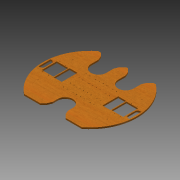
# Autodesk Inventor part: ChassisRound
Saved by Autodesk Inventor 2014 SP1 (Build 180222100, 222)
## iProperties
Created: 2015-03-16
Part Number: ChassisRound
Material: Wood (Oak)
Document SubType Name: Modeling
Designer: david
Density: 0.76 g/cm^3
Appearance: Yellow Pine - Solid Stained Light Low Gloss
Mass: 358.304 g
Surface Area: 1717.54 cm^2
Volume: 471.453 cm^3
Chassis_Body_Length: 300,000 mm
Chassis_Body_Diameter: 380,000 mm
Chassis_Body_Thickness: 6,000 mm
Author: david
Autodesk Inventor part; units mm, degrees
ref_plane "YZ Plane" through (0, 0, 0) normal (1, 0, 0) x (0, 1, 0)
ref_plane "XZ Plane" through (0, 0, 0) normal (0, 1, 0) x (-1, 0, 0)
ref_plane "XY Plane" through (0, 0, 0) normal (0, 0, 1) x (1, 0, 0)
sketch "BodySketch" plane through (0, 0, 0) normal (0, 1, 0) x (-1, 0, 0)
  line L0 (0, 150) -> (116.619, 150)
  line L1 (116.619, -150) -> (0, -150)
  line L2 (0, 0) -> (0, 145.614) construction
  line L3 (0, 150) -> (-116.619, 150)
  line L4 (-116.619, -150) -> (0, -150)
  line L5 (0, 0) -> (316.974, 0) construction
  arc A0 (116.619, -150) -> (116.619, 150) centre (0, 0) ccw
  arc A1 (-116.619, 150) -> (-116.619, -150) centre (0, 0) ccw
  dimension "Chassis_Body_Length" = 300
  dimension "d76" = 190
  constraints: 12 end point, 4 point on circle, 3 parallel, 2 centre point, 2 point on line, 2 symmetric about line, 1 coincident, 1 horizontal, 1 perpendicular, 1 other
  measures "Chassis_Body_Length" distance between parallel lines of L1 L0
  measures "d76" radius of A0
extrude "Body" add sketch "BodySketch" along normal blind 6
sketch "EncoderWheelHoleSketch" plane through (0, 6, 0) normal (0, 1, 0) x (1, 0, 0)
  line L0 (-168.5, 18) -> (-168.5, -18)
  line L1 (-184, -24.5) -> (-184, 24.5)
  line L2 (-116.619, -150) -> (116.619, -150) projected
  arc A0 (-116.619, 150) -> (-116.619, -150) centre (0, 0) ccw projected
  line L3 (-184, 24.5) -> (-177, 24.5)
  line L4 (-177, 24.5) -> (-168.5, 18)
  line L5 (-168.5, -18) -> (-177, -24.5)
  line L6 (-177, -24.5) -> (-184, -24.5)
  line L7 (0, 0) -> (-101.7765, 0) construction
  line L8 (0, 0) -> (0, 68.8757) construction
  line L9 (168.5, 18) -> (168.5, -18)
  line L10 (184, -24.5) -> (184, 24.5)
  line L11 (184, 24.5) -> (177, 24.5)
  line L12 (177, 24.5) -> (168.5, 18)
  line L13 (168.5, -18) -> (177, -24.5)
  line L14 (177, -24.5) -> (184, -24.5)
  point P0 (-190, 0)
  dimension "d80" = 7
  dimension "d81" = 15.5
  dimension "d82" = 49
  dimension "d83" = 36
  dimension "d84" = 6
  constraints: 28 end point, 7 symmetric about line, 5 parallel, 1 perpendicular, 1 point on circle, 1 point on line, 1 other
  measures "d80" distance of L1.end L3.end
  measures "d81" distance between parallel lines of L0 L1
  measures "d82" distance between parallel lines of L6 L3
  measures "d83" distance of L0.start L0.end
  measures "d84" distance from line of point (-190, 0) L1
extrude "EncoderWheelHole" cut sketch "EncoderWheelHoleSketch" against normal up to next
sketch "EncoderBodyHoleSketch" plane through (0, 6, 0) normal (0, 1, 0) x (1, 0, 0)
  line L0 (0, 0) -> (0, 145.3586) construction
  line L1 (-164.5, 30.25) -> (-117.5, 30.25)
  line L2 (-117.5, 30.25) -> (-117.5, -30.25)
  line L3 (-117.5, -30.25) -> (-164.5, -30.25)
  line L4 (-164.5, -30.25) -> (-164.5, 30.25)
  line L5 (0, 0) -> (187.4589, 0) construction
  line L6 (164.5, 30.25) -> (117.5, 30.25)
  line L7 (117.5, 30.25) -> (117.5, -30.25)
  line L8 (117.5, -30.25) -> (164.5, -30.25)
  line L9 (164.5, -30.25) -> (164.5, 30.25)
  line L10 (-141, -22.1441) -> (-141, 50.5352) construction
  line L11 (-168.5, 18) -> (-168.5, -18) projected
  line L12 (-184, -24.5) -> (-184, 24.5) projected
  dimension "d9" = 47
  dimension "d10" = 60.5
  dimension "d85" = 43
  constraints: 22 end point, 4 symmetric about line, 3 parallel, 2 perpendicular, 1 horizontal, 2 other
  measures "d9" distance between parallel lines of L2 L4
  measures "d10" distance between parallel lines of L3 L1
  measures "d85" distance between parallel lines of L12 L10
extrude "EncoderBodyHole" cut sketch "EncoderBodyHoleSketch" against normal up to next
sketch "EncoderSupportFasteningSketch" plane through (0, 6, 0) normal (0, 1, 0) x (1, 0, 0)
  line L0 (-128.5, 39.75) -> (-161.5, 39.75) construction
  line L1 (-161.5, 39.75) -> (-161.5, -39.75) construction
  line L2 (-128.5, -39.75) -> (-128.5, 39.75) construction
  circle A0 centre (-156.5, 34.75) radius 1.5
  line L3 (-145, 46.4919) -> (-145, -51.9033) construction
  circle A1 centre (-133.5, 34.75) radius 1.5
  line L4 (0, 0) -> (78.2402, 0) construction
  circle A2 centre (-156.5, -34.75) radius 1.5
  circle A3 centre (-133.5, -34.75) radius 1.5
  line L5 (-161.5, -39.75) -> (-128.5, -39.75) construction
  line L6 (0, 0) -> (0, 64.4845) construction
  circle A4 centre (156.5, 34.75) radius 1.5
  circle A5 centre (133.5, 34.75) radius 1.5
  circle A6 centre (156.5, -34.75) radius 1.5
  circle A7 centre (133.5, -34.75) radius 1.5
  line L7 (-184, -24.5) -> (-184, 24.5) projected
  dimension "d17" = 33
  dimension "d19" = 3
  dimension "d20" = 5
  dimension "d21" = 5
  dimension "d22" = 16.5
  dimension "d69" = 79.5
  dimension "d86" = 22.5
  constraints: 14 end point, 8 centre point, 7 symmetric about line, 2 parallel, 2 perpendicular, 1 horizontal, 8 other
  measures "d17" distance between parallel lines of L1 L2
  measures "d19" diameter of A0
  measures "d20" distance from line of L0 A0.centre
  measures "d21" distance from line of L1 A0.centre
  measures "d22" distance between parallel lines of L1 L3
  measures "d69" distance between parallel lines of L5 L0
  measures "d86" distance between parallel lines of L7 L1
extrude "EncoderSupportFastening" cut sketch "EncoderSupportFasteningSketch" against normal up to next
sketch "MotorBlockFasteningSketch" plane through (0, 6, 0) normal (0, 1, 0) x (1, 0, 0)
  line L0 (10.676, -18) -> (24.3135, -18) construction
  circle A0 centre (7.5, -18) radius 1.5
  circle A1 centre (22.5, -18) radius 1.5
  line L1 (0, 0) -> (0, -28.6489) construction
  circle A2 centre (46.5, -18) radius 1.5
  circle A3 centre (61.5, -18) radius 1.5
  circle A4 centre (7.5, -46) radius 1.5
  circle A5 centre (22.5, -46) radius 1.5
  circle A6 centre (46.5, -46) radius 1.5
  circle A7 centre (61.5, -46) radius 1.5
  circle A8 centre (-7.5, -18) radius 1.5
  circle A9 centre (-22.5, -18) radius 1.5
  circle A10 centre (-46.5, -18) radius 1.5
  circle A11 centre (-61.5, -18) radius 1.5
  circle A12 centre (-7.5, -46) radius 1.5
  circle A13 centre (-22.5, -46) radius 1.5
  circle A14 centre (-46.5, -46) radius 1.5
  circle A15 centre (-61.5, -46) radius 1.5
  line L2 (0, 0) -> (72.0385, 0) construction
  circle A16 centre (7.5, 18) radius 1.5
  circle A17 centre (22.5, 18) radius 1.5
  line L3 (0, 0) -> (0, 28.6489) construction
  circle A18 centre (46.5, 18) radius 1.5
  circle A19 centre (61.5, 18) radius 1.5
  circle A20 centre (7.5, 46) radius 1.5
  circle A21 centre (22.5, 46) radius 1.5
  circle A22 centre (46.5, 46) radius 1.5
  circle A23 centre (61.5, 46) radius 1.5
  circle A24 centre (-7.5, 18) radius 1.5
  circle A25 centre (-22.5, 18) radius 1.5
  circle A26 centre (-46.5, 18) radius 1.5
  circle A27 centre (-46.5, 46) radius 1.5
  circle A28 centre (-61.5, 18) radius 1.5
  circle A29 centre (-61.5, 46) radius 1.5
  circle A30 centre (-7.5, 46) radius 1.5
  circle A31 centre (-22.5, 46) radius 1.5
  dimension "d25" = 3
  dimension "d28" = 15
  dimension "d35" = 39
  dimension "d38" = 28
  dimension "d41" = 15
  dimension "d46" = 18
  constraints: 32 centre point, 25 symmetric about line, 8 end point, 3 horizontal, 1 perpendicular, 1 point on line, 1 vertical, 38 other
  measures "d25" diameter of A0
  measures "d28" distance of A0.centre A1.centre
  measures "d35" distance of A0.centre A2.centre
  measures "d38" distance of A0.centre A4.centre
  measures "d41" distance of A0.centre A8.centre
  measures "d46" distance between parallel lines of L2 L0
extrude "MotorBlockFastening" cut sketch "MotorBlockFasteningSketch" against normal up to next
sketch "MotorWheelHoleSketch" plane through (0, 6, 0) normal (0, 1, 0) x (1, 0, 0)
  line L0 (-114.5, 32) -> (-82.5, 32)
  line L1 (-82.5, 32) -> (-82.5, -32)
  line L2 (-82.5, -32) -> (-114.5, -32)
  line L3 (-114.5, -32) -> (-114.5, 32)
  line L4 (0, 0) -> (64.8732, 0) construction
  line L5 (0, 0) -> (0, 63.2492) construction
  line L6 (-117.5, 30.25) -> (-117.5, -30.25) construction
  line L7 (114.5, 32) -> (82.5, 32)
  line L8 (82.5, 32) -> (82.5, -32)
  line L9 (82.5, -32) -> (114.5, -32)
  line L10 (114.5, -32) -> (114.5, 32)
  dimension "Chassis_MotorWheelHole_Diameter" = 64
  dimension "Chassis_MotorWheelHole_Width" = 32
  dimension "Chassis_MotorWheelHole_DistanceToEncoder" = 3
  constraints: 20 end point, 4 symmetric about line, 3 perpendicular, 2 parallel, 1 horizontal, 1 other
  measures "Chassis_MotorWheelHole_Diameter" distance between parallel lines of L2 L0
  measures "Chassis_MotorWheelHole_Width" distance between parallel lines of L1 L3
  measures "Chassis_MotorWheelHole_DistanceToEncoder" distance between parallel lines of L6 L3
extrude "MotorWheelHole" cut sketch "MotorWheelHoleSketch" against normal up to next
sketch "Sketch11" plane through (0, 6, 0) normal (0, 1, 0) x (1, 0, 0)
  line L0 (-116.619, -150) -> (116.619, -150) projected
  arc A0 (116.619, -150) -> (116.619, 150) centre (0, 0) ccw projected
  line L1 (116.619, 150) -> (-116.619, 150) projected
  arc A1 (-116.619, 150) -> (-116.619, -150) centre (0, 0) ccw projected
  arc A2 (31, -100) -> (-31, -100) centre (0, -100) ccw
  line L2 (0, 0) -> (0, -208.4232) construction
  line L3 (-31, -100) -> (-31, -150)
  line L4 (31, -100) -> (31, -150)
  dimension "d88" = 31
  dimension "d90" = 100
  constraints: 6 end point, 3 point on line, 2 perpendicular, 2 point on circle, 2 tangent, 1 centre point, 1 parallel
  measures "d88" radius of A2
  measures "d90" distance of A0.centre A2.centre
extrude "StandHole" cut sketch "Sketch11" against normal up to next contours L3 A2 L4 L0
sketch "Sketch12" plane through (0, 6, 0) normal (0, 1, 0) x (1, 0, 0)
  line L0 (116.619, 150) -> (-116.619, 150) projected
  arc A0 (-116.619, 150) -> (-116.619, -150) centre (0, 0) ccw projected
  line L1 (-82.5, -32) -> (-114.5, -32) projected
  arc A1 (-86, 90) -> (-24, 90) centre (-55, 90) ccw
  line L2 (0, 0) -> (0, 75.9488) construction
  arc A2 (24, 90) -> (86, 90) centre (55, 90) ccw
  circle A3 centre (-55, 90) radius 50 construction
  circle A4 centre (55, 90) radius 50 construction
  line L3 (-86, 90) -> (-86, 150)
  line L4 (-24, 90) -> (-24, 150)
  line L5 (24, 90) -> (24, 150)
  line L6 (86, 90) -> (86, 150)
  dimension "d93" = 62
  dimension "d94" = 100
  dimension "d95" = 100
  dimension "d96" = 110
  dimension "d97" = 60
  constraints: 10 end point, 4 centre point, 4 perpendicular, 4 point on circle, 4 point on line, 4 tangent, 2 coincident, 1 parallel, 1 symmetric about line, 1 other
  measures "d93" diameter of A1
  measures "d94" diameter of A3
  measures "d95" diameter of A4
  measures "d96" distance of A4.centre A3.centre
  measures "d97" distance from line of L0 A1.centre
extrude "PopcornCupHoles" cut sketch "Sketch12" against normal up to next
chamfer "PlayingElementHoleGuide1" distance 20 angle 45 6 edges at (-86, 3, -150) (24, 3, -150) (86, 3, -150) (-24, 3, -150) (-31, 3, 150) (31, 3, 150)
chamfer "PlayingElementHoleGuide2" distance 10 angle 45 6 edges at (-86, 3, -130) (-24, 3, -130) (24, 3, -130) (86, 3, -130) (-31, 3, 130) (31, 3, 130)
sketch "StructureColumnHolesSketch" plane through (0, 6, 0) normal (0, 1, 0) x (1, 0, 0)
  arc A0 (-116.619, 150) -> (-116.619, -150) centre (0, 0) ccw projected
  line L0 (-148.5, 61.5) -> (-131.5, 61.5) construction
  line L1 (-131.5, 61.5) -> (-131.5, 78.5) construction
  line L2 (-131.5, 78.5) -> (-148.5, 78.5) construction
  line L3 (-148.5, 78.5) -> (-148.5, 61.5) construction
  line L4 (-148.5, 61.5) -> (-131.5, 78.5) construction
  line L5 (-131.5, 61.5) -> (-148.5, 78.5) construction
  circle A1 centre (-140, 70) radius 1.5
  line L6 (0, 0) -> (0, 92.1704) construction
  line L7 (0, 0) -> (226.7132, 0) construction
  line L8 (148.5, 61.5) -> (131.5, 61.5) construction
  line L9 (131.5, 61.5) -> (131.5, 78.5) construction
  line L10 (131.5, 78.5) -> (148.5, 78.5) construction
  line L11 (148.5, 78.5) -> (148.5, 61.5) construction
  circle A2 centre (140, 70) radius 1.5
  line L12 (-148.5, -61.5) -> (-131.5, -61.5) construction
  line L13 (-131.5, -61.5) -> (-131.5, -78.5) construction
  line L14 (-131.5, -78.5) -> (-148.5, -78.5) construction
  line L15 (-148.5, -78.5) -> (-148.5, -61.5) construction
  circle A3 centre (-140, -70) radius 1.5
  circle A4 centre (140, -70) radius 1.5
  line L16 (131.5, -61.5) -> (131.5, -78.5) construction
  line L17 (131.5, -78.5) -> (148.5, -78.5) construction
  line L18 (148.5, -78.5) -> (148.5, -61.5) construction
  line L19 (148.5, -61.5) -> (131.5, -61.5) construction
  dimension "d106" = 17
  dimension "d107" = 17
  dimension "d108" = 3
  dimension "d111" = 280
  dimension "d112" = 140
  constraints: 40 end point, 15 symmetric about line, 4 centre point, 3 parallel, 2 midpoint, 2 perpendicular, 1 coincident, 1 horizontal, 3 other
  measures "d106" distance of L2.end L1.end
  measures "d107" distance of L1.end L0.end
  measures "d108" diameter of A1
  measures "d111" distance of A2.centre point (-140, 70)
  measures "d112" distance of A4.centre A2.centre
extrude "StructureColumnHoles" cut sketch "StructureColumnHolesSketch" against normal up to next
equation "\"d10\" = EncoderSupportInside_Width + 2 * Chassis_MecanicalSpace"
equation "\"d17\" = EncoderSupportOutside_Length"
equation "\"d19\" = EncoderSupport_FixingHole_Diameter"
equation "\"d20\" = EncoderSupport_FixingnHole_Margin"
equation "\"d21\" = EncoderSupport_FixingnHole_Margin"
equation "\"d22\" = 0.5 * EncoderSupportOutside_Length"
equation "\"d28\" = Bracket_Holes_Distance"
equation "\"d35\" = Bracket_Holes_Distance + Bracket_Holes_UnfoldedDistance"
equation "\"d38\" = Bracket_Holes_LateralDistance"
equation "\"d41\" = Bracket_Holes_Distance"
equation "\"d46\" = Motor_FasteningHole_DistanceToCenter"
equation "\"Chassis_MecanicalSpace\" = 1"
equation "\"EncoderSupportInside_Width\" = 58.5"
equation "\"EncoderSupportOutside_Length\" = 33"
equation "\"EncoderSupport_FixingHole_Diameter\" = 3"
equation "\"EncoderSupport_FixingnHole_Margin\" = 5"
equation "\"Bracket_Holes_Distance\" = 15"
equation "\"Bracket_Holes_UnfoldedDistance\" = 24"
equation "\"Bracket_Holes_LateralDistance\" = 28"
equation "\"Motor_FasteningHole_DistanceToCenter\" = 18"
body "Solid1"
